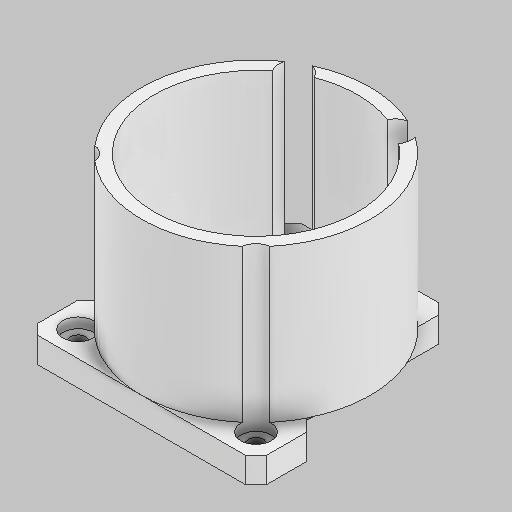
# Autodesk Inventor part: top plate
Saved by Autodesk Inventor 2025.2 (Build 292293000, 293)
## iProperties
Created: 2025-03-25
Part Number: top plate
Material: PC/ABS Plastic
Document SubType Name: Modeling
Designer: joaki
Density: 1.1 g/cm^3
Appearance: Smooth - White
Mass: 17.8175 g
Surface Area: 122.713 cm^2
Volume: 16.1978 cm^3
Author: joaki
Autodesk Inventor part; units mm, degrees
ref_plane "YZ Plane" through (0, 0, 0) normal (1, 0, 0) x (0, 1, 0)
ref_plane "XZ Plane" through (0, 0, 0) normal (0, 1, 0) x (-1, 0, 0)
ref_plane "XY Plane" through (0, 0, 0) normal (0, 0, 1) x (1, 0, 0)
sketch "Sketch1" plane through (0, 0, 0) normal (0, 1, 0) x (-1, 0, 0)
  line L0 (13.0677, 24.5961) -> (-31.9323, 24.5961)
  line L1 (-31.9323, 24.5961) -> (-31.9323, -20.4039)
  line L2 (-31.9323, -20.4039) -> (13.0677, -20.4039)
  line L3 (13.0677, -20.4039) -> (13.0677, 24.5961)
  line L4 (-9.4323, 24.5961) -> (-9.4323, -20.4039)
  circle A0 centre (-26.9323, 19.5961) radius 1.5
  circle A1 centre (8.0677, 19.5961) radius 1.5
  circle A2 centre (0.5677, -15.4039) radius 1.5
  circle A3 centre (-19.4323, -15.4039) radius 1.5
  line L5 (-9.4323, -6.949) -> (6.0677, -6.949)
  line L6 (13.0677, 24.5961) -> (13.0677, 8.5961)
  line L7 (13.0677, 8.5961) -> (6.0677, 8.5961)
  line L8 (6.0677, 8.5961) -> (6.0677, -20.4039)
  line L9 (13.0677, 24.5961) -> (13.0677, 14.5961)
  line L10 (13.0677, 14.5961) -> (6.0677, 14.5961)
  line L11 (6.0677, 14.5961) -> (6.0677, 8.5961)
  line L12 (-31.9323, 24.5961) -> (-31.9323, 14.5961)
  line L13 (-31.9323, 14.5961) -> (-24.9323, 14.5961)
  line L14 (-24.9323, 14.5961) -> (-24.9323, -20.4039)
  line L15 (13.0677, 14.5961) -> (13.0677, 7.5961)
  line L16 (13.0677, 7.5961) -> (6.0677, 7.5961)
  line L17 (-31.9323, 14.5961) -> (-31.9323, 7.5961)
  line L18 (-31.9323, 7.5961) -> (-24.9323, 7.5961)
  point P0 (0, 0)
  dimension "d0" = 45
  dimension "d1" = 45
  dimension "d2" = 3
  dimension "d3" = 3
  dimension "d4" = 35
  dimension "d5" = 5
  dimension "d6" = 5
  dimension "d7" = 5
  dimension "d8" = 5
  dimension "d9" = 3
  dimension "d10" = 3
  dimension "d11" = 20
  dimension "d12" = 5
  dimension "d13" = 5
  dimension "d14" = 10
  dimension "d15" = 15.5
  dimension "d16" = 16
  dimension "d17" = 10
  dimension "d18" = 10
  dimension "d19" = 7
  dimension "d20" = 7
  dimension "d26" = 7
  dimension "d27" = 7
  constraints: 38 end point, 11 point on line, 9 perpendicular, 4 centre point, 2 horizontal, 2 midpoint, 2 parallel
  measures "d0" distance of L2.end L0.start
  measures "d1" distance of L1.end L2.end
  measures "d2" diameter of A0
  measures "d3" diameter of A1
  measures "d4" distance of A0.centre A1.centre
  measures "d5" distance from line of L0 A1.centre
  measures "d6" distance from line of L3 A1.centre
  measures "d7" distance from line of L0 A0.centre
  measures "d8" distance from line of L1 A0.centre
  measures "d9" diameter of A2
  measures "d10" diameter of A3
  measures "d11" distance of A2.centre A3.centre
  measures "d12" distance from line of L2 A2.centre
  measures "d13" distance from line of L2 A3.centre
  measures "d14" distance from line of L4 A3.centre
  measures "d15" distance of L5.start L5.end
  measures "d16" distance of L0.start L6.end
  measures "d17" distance of L0.start L9.end
  measures "d18" distance of L0.end L12.end
  measures "d19" distance between parallel lines of L3 L8
  measures "d20" distance of L12.end L13.end
  measures "d26" distance of L9.end L15.end
  measures "d27" distance of L12.end L17.end
extrude "Extrusion1" add sketch "Sketch1" along normal blind 3 contours L3 L10 L11 L8 L5 L4 L0 | L4 L2 L14 L13 L1 L0 | L3 L7 L11 L10 | L5 L8 L2 L4 | L3 L16 L8 L7 | L13 L14 L18 L1
chamfer "Chamfer1" distance 2 angle 45 4 edges at (31.9323, 1.5, 24.5961) (24.9323, 1.5, -20.4039) (-6.0677, 1.5, -20.4039) (-13.0677, 1.5, 24.5961)
chamfer "Chamfer2" distance 7 angle 45 2 edges at (31.9323, 1.5, 7.5961) (-13.0677, 1.5, 7.5961)
sketch "Sketch5" plane through (0, 3, 0) normal (0, 1, 0) x (1, 0, 0)
  line L0 (-11.0677, -24.5961) -> (29.9323, -24.5961) projected
  line L1 (9.4323, -24.5961) -> (9.4323, 20.4039)
  line L2 (22.9323, 20.4039) -> (-4.0677, 20.4039) projected
  circle A0 centre (26.9323, -19.5961) radius 1.5 projected
  circle A1 centre (26.9323, -19.5961) radius 3
  circle A2 centre (-8.0677, -19.5961) radius 1.5 projected
  circle A3 centre (-8.0677, -19.5961) radius 3
  circle A4 centre (-0.5677, 15.4039) radius 1.5 projected
  circle A5 centre (-0.5677, 15.4039) radius 3
  circle A6 centre (19.4323, 15.4039) radius 1.5 projected
  circle A7 centre (19.4323, 15.4039) radius 3
  line L3 (31.9323, -22.5961) -> (31.9323, -14.5961) projected
  line L4 (31.9323, -22.5961) -> (29.9323, -24.5961)
  line L5 (-11.0677, -24.5961) -> (-13.0677, -22.5961)
  line L6 (-13.0677, -22.5961) -> (-13.0677, -14.5961)
  line L7 (-13.0677, -14.5961) -> (-6.5677, -8.0961)
  line L8 (-6.0677, 18.4039) -> (-6.0677, -7.5961) projected
  line L9 (-6.5677, -8.0961) -> (-6.0677, -7.5961)
  line L10 (-6.0677, -7.5961) -> (-6.0677, 18.4039)
  line L11 (-6.0677, 18.4039) -> (-4.0677, 20.4039)
  line L12 (22.9323, 20.4039) -> (-4.0677, 20.4039)
  line L13 (22.9323, 20.4039) -> (24.9323, 18.4039)
  line L14 (24.9323, 18.4039) -> (24.9323, -7.5961)
  line L15 (24.9323, -7.5961) -> (31.9323, -14.5961)
  point P0 (0, 0)
  dimension "d59" = 6
  dimension "d60" = 6
  dimension "d61" = 6
  dimension "d62" = 6
  constraints: 24 end point, 5 perpendicular, 4 centre point, 4 coincident, 3 parallel, 2 collinear, 2 midpoint
  measures "d59" diameter of A1
  measures "d60" diameter of A3
  measures "d61" diameter of A5
  measures "d62" diameter of A7
extrude "Extrusion5" add sketch "Sketch5" along normal blind 2 contours L5 L6 L7 L9 L8 L11 L2 L1 L0 | L1 L2 L13 L14 L15 L3 L4 L0
sketch "Sketch6" plane through (0, 5, 0) normal (0, 1, 0) x (1, 0, 0)
  line L0 (-11.0677, -24.5961) -> (29.9323, -24.5961) projected
  line L1 (9.4323, -24.5961) -> (9.4323, 20.4039)
  line L2 (22.9323, 20.4039) -> (-4.0677, 20.4039) projected
  circle A0 centre (9.4323, -2.0961) radius 20
  circle A1 centre (9.4323, -2.0961) radius 22.5
  line L3 (31.9323, -14.5961) -> (24.9323, -7.5961) projected
  line L4 (27.6611, -10.3248) -> (29.5361, -12.1999)
  line L5 (-8.7964, -10.3248) -> (-10.6715, -12.1999)
  line L6 (-6.0677, -7.5961) -> (-13.0677, -14.5961) projected
  line L7 (-6.0677, 14.2134) -> (-6.0677, 10.5432)
  line L8 (-6.0677, 18.4039) -> (-6.0677, -7.5961) projected
  line L9 (24.9323, 14.2134) -> (24.9323, 10.5432)
  line L10 (24.9323, -7.5961) -> (24.9323, 18.4039) projected
  circle A2 centre (19.4323, 15.4039) radius 3 projected
  circle A3 centre (19.4323, 15.4039) radius 3
  circle A4 centre (-0.5677, 15.4039) radius 3 projected
  circle A5 centre (-0.5677, 15.4039) radius 3
  circle A6 centre (-8.0677, -19.5961) radius 3 projected
  circle A7 centre (-8.0677, -19.5961) radius 3
  circle A8 centre (26.9323, -19.5961) radius 1.5 projected
  circle A9 centre (26.9323, -19.5961) radius 3
  point P0 (0, 0)
  point P1 (0.0278, 18.3442)
  point P2 (2.2039, 16.552)
  point P3 (16.6607, 16.552)
  point P4 (18.8368, 18.3442)
  point P5 (23.9482, -19.2873)
  point P6 (26.6235, -16.612)
  point P7 (22.2678, 16.3836)
  point P8 (21.8286, 13.5989)
  point P9 (-2.9639, 13.5989)
  point P10 (-3.4032, 16.3836)
  point P11 (-7.7589, -16.612)
  point P12 (-5.0836, -19.2873)
  dimension "d65" = 40
  constraints: 10 end point, 9 point on circle, 6 centre point, 5 coincident, 5 point on line, 3 midpoint
  measures "d65" diameter of A0
extrude "Extrusion6" add sketch "Sketch6" along normal blind 30 contours A1 A6 L5 A0 L1 | L1 A0 L3 A1 A9 | A0 A4 A1 L1 | L1 A1 A2 A0 | L5 A1 L7 A0 | A0 L9 A1 L3 | L7 A1 A4 A0 | A2 A1 L9 A0
sketch "Sketch7" plane through (0, 5, 0) normal (0, 1, 0) x (1, 0, 0)
  arc A0 (-2.9639, 13.5989) -> (21.8286, 13.5989) centre (9.4323, -2.0961) ccw projected
  circle A1 centre (9.4323, -2.0961) radius 20
  line L0 (9.4323, 17.9039) -> (9.4323, -6.0961)
  line L1 (9.4323, -6.0961) -> (-0.0677, -6.0961)
  line L2 (-0.0677, -6.0961) -> (18.9323, -6.0961)
  line L3 (18.9323, -6.0961) -> (18.9323, 15.5036)
  line L4 (-0.0677, -6.0961) -> (-0.0677, 15.5036)
  line L5 (-0.0677, -6.0961) -> (-6.0677, -6.0961)
  line L6 (-6.0677, 18.4039) -> (-6.0677, -7.5961) projected
  line L7 (-6.0677, -6.0961) -> (-6.0677, 10.5432)
  line L8 (18.9323, -6.0961) -> (24.9323, -6.0961)
  line L9 (24.9323, -7.5961) -> (24.9323, 18.4039) projected
  line L10 (24.9323, -6.0961) -> (24.9323, 10.5432)
  point P0 (0, 0)
  point P1 (-6.0677, 10.5432)
  point P2 (-2.9639, 13.5989)
  point P3 (24.9323, 10.5432)
  point P4 (21.8286, 13.5989)
  dimension "d68" = 24
  dimension "d69" = 9.5
  dimension "d70" = 19
  constraints: 18 end point, 7 point on line, 5 point on circle, 2 perpendicular, 1 centre point, 1 coincident, 1 parallel, 1 vertical
  measures "d68" distance of L0.start L0.end
  measures "d69" distance of L0.end L1.end
  measures "d70" distance of L1.end L2.end
extrude "Extrusion7" cut sketch "Sketch7" against normal blind 2 contours A1 L4 L5 L6 A0 | L9 L8 L3 A1 A0
body "Solid1"
